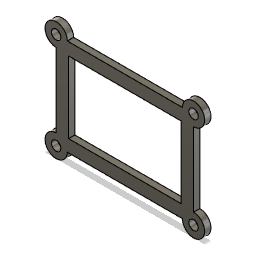
Beam_Split_Bracket_top v2 (Autodesk Fusion 360 design; units mm, degrees)
Autodesk Fusion 360 part; units mm, degrees
sketch "Sketch1" plane through (0, 0, 0) normal (0, 0, 1) x (1, 0, 0)
  line L0 (5, 65) -> (43.5, 65)
  line L1 (43.5, 65) -> (43.5, 39.5)
  line L2 (43.5, 39.5) -> (5, 39.5)
  line L3 (5, 39.5) -> (5, 65)
  line L4 (5, 65) -> (5, 67.5)
  line L5 (5, 67.5) -> (2.5, 67.5)
  line L6 (2.5, 67.5) -> (2.5, 37)
  line L7 (2.5, 37) -> (3, 37)
  line L8 (3, 37) -> (46, 37)
  line L9 (46, 37) -> (46, 67.5)
  line L10 (46, 67.5) -> (5, 67.5)
  dimension "d1" = 38.5
  dimension "d2" = 25.5
  dimension "d3" = 2.5
  dimension "d4" = 2.5
  dimension "d5" = 30.5
  dimension "d6" = 43
  constraint horizontal L0
  constraint vertical L1
  constraint horizontal L2
  constraint vertical L3
  constraint perpendicular L0 L4
  constraint perpendicular L4 L5
  constraint perpendicular L2 L6
  constraint perpendicular L6 L7
  constraint perpendicular L6 L8
  constraint perpendicular L5 L9
  constraint perpendicular L4 L10
  measures "d1" distance of L0.start L0.end
  measures "d2" distance of L0.start L2.end
  measures "d3" distance of L0.start L4.end
  measures "d4" distance of L4.end L5.end
  measures "d5" distance of L5.end L6.end
  measures "d6" distance of L7.end L8.end
extrude "Extrude1" add sketch "Sketch1" along normal blind 3
sketch "Sketch2" plane through (0, 0, 3) normal (0, 0, 1) x (1, 0, 0)
  line L0 (43.5, 39.5) -> (5, 39.5)
  line L1 (5, 39.5) -> (5, 65)
  line L2 (5, 65) -> (43.5, 65)
  line L3 (43.5, 65) -> (43.5, 39.5)
  line L4 (46, 67.5) -> (2.5, 67.5)
  line L5 (2.5, 67.5) -> (2.5, 37)
  line L6 (2.5, 37) -> (46, 37)
  line L7 (46, 37) -> (46, 67.5)
  circle A0 centre (2.5, 67.5) radius 3.5355
  circle A1 centre (46, 67.5) radius 3.5355
  circle A2 centre (46, 37) radius 3.5355
  circle A3 centre (2.5, 37) radius 3.5355
  constraint coincident L4.end L5.start
  constraint coincident L1.end A0
  constraint coincident L4.start L7.end
  constraint coincident L2.end A1
  constraint coincident L6.end L7.start
  constraint coincident L0.start A2
  constraint coincident L5.end L6.start
  constraint coincident L0.end A3
extrude "Extrude2" add sketch "Sketch2" against normal blind 3 contours L6 L7 A2 | L5 L6 A3 | L4 L7 A1 | L4 L5 A0 picked at (43.6561, 36.8244) picked at (4.8443, 36.8271) picked at (43.6561, 67.6756) picked at (2.3271, 65.1557)
sketch "Sketch3" plane through (0, 0, 3) normal (0, 0, 1) x (1, 0, 0)
  line L0 (43.5, 39.5) -> (5, 39.5)
  line L1 (5, 39.5) -> (5, 65)
  line L2 (5, 65) -> (43.5, 65)
  line L3 (43.5, 65) -> (43.5, 39.5)
  line L4 (42.4645, 67.5) -> (6.0355, 67.5)
  arc A0 (6.0355, 67.5) -> (2.5, 63.9645) centre (2.5, 67.5) ccw
  line L5 (2.5, 63.9645) -> (2.5, 40.5355)
  arc A1 (2.5, 40.5355) -> (6.0355, 37) centre (2.5, 37) ccw
  line L6 (6.0355, 37) -> (42.4645, 37)
  arc A2 (42.4645, 37) -> (46, 40.5355) centre (46, 37) ccw
  line L7 (46, 40.5355) -> (46, 63.9645)
  arc A3 (46, 63.9645) -> (42.4645, 67.5) centre (46, 67.5) ccw
  circle A4 centre (2.5, 67.5) radius 1.5
  circle A5 centre (46, 67.5) radius 1.5
  circle A6 centre (2.5, 37) radius 1.5
  circle A7 centre (46, 37) radius 1.5
  dimension "d11" = 3
  dimension "d12" = 3
  dimension "d13" = 3
  dimension "d14" = 3
  constraint concentric A0 A4
  constraint concentric A3 A5
  constraint concentric A1 A6
  constraint concentric A2 A7
  measures "d11" diameter of A4
  measures "d12" diameter of A5
  measures "d13" diameter of A6
  measures "d14" diameter of A7
extrude "Extrude3" cut sketch "Sketch3" against normal blind 6 contours A4 | A5 | A6 | A7
extrude "Extrude4" add 1 faces at (18.1785, 38.6667, 3) along direction (0, 0, 1) blind 0.1
sketch "Sketch4" plane through (0, 0, 3.1) normal (0, 0, 1) x (1, 0, 0)
  circle A0 centre (2.5, 37) radius 1.5
  circle A1 centre (46, 67.5) radius 1.5
  circle A2 centre (2.5, 67.5) radius 1.5
  circle A3 centre (46, 37) radius 1.5
  line L0 (43.5, 39.5) -> (5, 39.5)
  line L1 (5, 39.5) -> (5, 65)
  line L2 (43.5, 65) -> (43.5, 39.5)
  line L3 (42.4645, 67.5) -> (6.0355, 67.5)
  arc A4 (6.0355, 67.5) -> (2.5, 63.9645) centre (2.5, 67.5) ccw
  line L4 (2.5, 63.9645) -> (2.5, 40.5355)
  arc A5 (2.5, 40.5355) -> (6.0355, 37) centre (2.5, 37) ccw
  line L5 (6.0355, 37) -> (42.4645, 37)
  arc A6 (42.4645, 37) -> (46, 40.5355) centre (46, 37) ccw
  line L6 (46, 40.5355) -> (46, 63.9645)
  arc A7 (46, 63.9645) -> (42.4645, 67.5) centre (46, 67.5) ccw
  circle A8 centre (2.5, 67.5) radius 3.5355
  circle A9 centre (46, 67.5) radius 3.5355
  circle A10 centre (2.5, 37) radius 3.5355
  circle A11 centre (46, 37) radius 3.5355
  line L7 (6.0355, 37) -> (42.4645, 37)
  line L8 (46, 40.5355) -> (46, 63.9645)
  line L9 (42.4645, 67.5) -> (6.0355, 67.5)
  line L10 (2.5, 63.9645) -> (2.5, 40.5355)
  line L11 (5, 65) -> (6.4142, 63.5858)
  line L12 (43.5, 65) -> (42.0858, 63.5858)
  line L13 (43.5, 65) -> (45.5, 65) construction
  line L14 (43.5, 39.5) -> (42.0858, 40.9142)
  line L15 (5, 39.5) -> (6.4142, 40.9142)
  line L16 (5, 39.5) -> (7, 39.5) construction
  line L17 (6.4142, 63.5858) -> (6.4142, 40.9142)
  line L18 (6.4142, 40.9142) -> (42.0858, 40.9142)
  line L19 (42.0858, 40.9142) -> (42.0858, 63.5858)
  line L20 (6.4142, 63.5858) -> (6.9321, 63.5858)
  line L21 (6.9321, 63.5858) -> (42.0858, 63.5858)
  dimension "d19" = 2
  dimension "d20" = 135
  dimension "d21" = 2
  dimension "d22" = 2
  dimension "d23" = 45
  dimension "d24" = 2
  constraint concentric A2 A8
  constraint concentric A1 A9
  constraint concentric A0 A10
  constraint concentric A3 A11
  constraint coincident A5.end L5.start
  constraint coincident L5.end A6.start
  constraint coincident A6.end L6.start
  constraint coincident L6.end A7.start
  constraint coincident L3.start A7.end
  constraint coincident L3.end A4.start
  constraint coincident A4.end L4.start
  constraint coincident L4.end A5.start
  constraint coincident L1.end L11.start
  constraint horizontal L13
  constraint coincident L2.start L12.start
  constraint coincident L0.start L2.end
  constraint horizontal L16
  constraint coincident L0.end L1.start
  constraint perpendicular L17 L20
  measures "d19" distance of L1.end L11.end
  measures "d20" angle of L12 L13
  measures "d21" distance of L2.start L12.end
  measures "d22" distance of L0.start L14.end
  measures "d23" angle of L15 L16
  measures "d24" distance of L0.end L15.end
extrude "Extrude5" add sketch "Sketch4" 1 faces at (18.1785, 38.6667, 3.1) along normal blind 1 contours L0 L5 A10 A11 L7 | L2 L12 L14 L19 | L2 L6 A9 A11 L8 | A6 A11 | L0 L14 L15 L18 | L1 L4 A8 A10 L10 | A5 A10 | L1 L11 L15 L17 | L3 A8 A9 L9 L11 L12 L20 L21 | A7 A9 | A4 A8
sketch "Sketch5" plane through (0, 37, 0) normal (0, -1, 0) x (1, 0, 0)
  line L0 (42.4645, 0) -> (42.4645, 4.1)
  line L1 (42.4645, 4.1) -> (6.0355, 4.1)
  line L2 (6.0355, 4.1) -> (6.0355, 0)
  line L3 (6.0355, 0) -> (42.4645, 0)
  line L4 (24.25, 0) -> (24.25, 1)
  line L5 (24.25, 1) -> (24.25, 4.1)
  line L6 (24.25, 4.1) -> (29.25, 4.1)
  line L7 (24.25, 4.1) -> (19.25, 4.1)
  line L8 (19.25, 4.1) -> (19.25, 0)
  line L9 (29.25, 4.1) -> (29.25, 0)
  line L10 (29.25, 0) -> (19.25, 0)
  dimension "d27" = 5
  dimension "d28" = 5
  constraint midpoint L3 L4.start
  constraint perpendicular L3 L4
  constraint midpoint L1 L5.end
  constraint perpendicular L3 L5
  constraint perpendicular L5 L6
  constraint perpendicular L5 L7
  constraint coincident L3 L8.end
  constraint perpendicular L3 L8
  constraint coincident L3 L9.end
  constraint perpendicular L3 L9
  measures "d27" distance of L5.end L6.end
  measures "d28" distance of L5.end L7.end
extrude "Extrude6" add sketch "Sketch5" along normal blind 10 contours L1 L3 L4 L5 L6 L9 L10 | L1 L3 L4 L5 L7 L8 L10
sketch "Sketch6" plane through (0, 0, 0) normal (0, 0, -1) x (-1, 0, 0)
  circle A0 centre (-2.5, 37) radius 1.5
  circle A1 centre (-46, 67.5) radius 1.5
  circle A2 centre (-2.5, 67.5) radius 1.5
  circle A3 centre (-46, 37) radius 1.5
  line L0 (-5, 39.5) -> (-43.5, 39.5)
  line L1 (-43.5, 39.5) -> (-43.5, 65)
  line L2 (-43.5, 65) -> (-5, 65)
  line L3 (-5, 65) -> (-5, 39.5)
  arc A4 (-42.4645, 67.5) -> (-46, 63.9645) centre (-46, 67.5) ccw
  line L4 (-46, 63.9645) -> (-46, 40.5355)
  arc A5 (-46, 40.5355) -> (-42.4645, 37) centre (-46, 37) ccw
  line L5 (-42.4645, 37) -> (-29.25, 37)
  line L6 (-29.25, 37) -> (-29.25, 27)
  line L7 (-29.25, 27) -> (-19.25, 27)
  line L8 (-19.25, 27) -> (-19.25, 37)
  line L9 (-19.25, 37) -> (-6.0355, 37)
  arc A6 (-6.0355, 37) -> (-2.5, 40.5355) centre (-2.5, 37) ccw
  line L10 (-2.5, 40.5355) -> (-2.5, 63.9645)
  arc A7 (-2.5, 63.9645) -> (-6.0355, 67.5) centre (-2.5, 67.5) ccw
  line L11 (-6.0355, 67.5) -> (-42.4645, 67.5)
  line L12 (-29.25, 27) -> (-29.25, 32)
  line L13 (-29.25, 32) -> (-19.25, 32)
  line L14 (-19.25, 32) -> (-19.25, 27)
  line L15 (-19.25, 27) -> (-29.25, 27)
  constraint coincident L6.end L7.start
  constraint midpoint L6 L12.end
  constraint midpoint L8 L13.end
  constraint coincident L7.end L8.start
extrude "Extrude7" add sketch "Sketch6" along normal blind 10 contours L6 L7 L8 L12 L13 L14 L15
sketch "Sketch7" plane through (0, 32, 0) normal (0, 1, 0) x (-1, 0, 0)
  line L0 (-19.25, 0) -> (-29.25, 0)
  line L1 (-29.25, 0) -> (-29.25, -10)
  line L2 (-29.25, -10) -> (-19.25, -10)
  line L3 (-19.25, -10) -> (-19.25, 0)
  line L4 (-24.25, -10) -> (-24.25, -5)
  circle A0 centre (-24.25, -5) radius 2
  dimension "d33" = 4
  constraint midpoint L2 L4.start
  constraint perpendicular L2 L4
  constraint coincident L4.end A0.centre
  measures "d33" diameter of A0
extrude "Extrude8" cut sketch "Sketch7" against normal blind 10 contours A0
extrude "Extrude9" cut 1 faces at (24.2002, 32, -1.0019) along direction (0, -1, 0) blind 11
sketch "Sketch8" plane through (0, 0, 0) normal (0, 0, -1) x (-1, 0, 0)
  line L0 (-19.25, 27) -> (-19.25, 37)
  line L1 (-19.25, 37) -> (-6.0355, 37)
  arc A0 (-6.0355, 37) -> (-2.5, 40.5355) centre (-2.5, 37) ccw
  line L2 (-2.5, 40.5355) -> (-2.5, 63.9645)
  arc A1 (-2.5, 63.9645) -> (-6.0355, 67.5) centre (-2.5, 67.5) ccw
  line L3 (-6.0355, 67.5) -> (-42.4645, 67.5)
  arc A2 (-42.4645, 67.5) -> (-46, 63.9645) centre (-46, 67.5) ccw
  line L4 (-46, 63.9645) -> (-46, 40.5355)
  arc A3 (-46, 40.5355) -> (-42.4645, 37) centre (-46, 37) ccw
  line L5 (-42.4645, 37) -> (-29.25, 37)
  line L6 (-29.25, 37) -> (-29.25, 27)
  line L7 (-29.25, 27) -> (-19.25, 27)
  circle A4 centre (-2.5, 37) radius 1.5
  circle A5 centre (-46, 67.5) radius 1.5
  circle A6 centre (-2.5, 67.5) radius 1.5
  circle A7 centre (-46, 37) radius 1.5
  line L8 (-5, 39.5) -> (-43.5, 39.5)
  line L9 (-43.5, 39.5) -> (-43.5, 65)
  line L10 (-43.5, 65) -> (-5, 65)
  line L11 (-5, 65) -> (-5, 39.5)
  line L12 (-29.25, 37) -> (-19.25, 37)
  constraint coincident L5.end L6.start
  constraint coincident L0.end L1.start
extrude "Extrude10" cut sketch "Sketch8" against normal blind 17 contours L0 L6 L7 L12
extrude "Extrude11" cut 1 faces at (18.1785, 38.6667, 0) along direction (0, 0, 1) blind 3.1
extrude "Extrude12" add 1 faces at (18.4774, 66.1953, 3.1) along direction (0, 0, -1) blind 1
